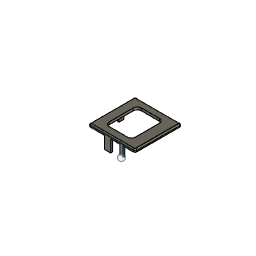
Lid (Autodesk Fusion 360 design; units mm, degrees)
Autodesk Fusion 360 part; units mm, degrees
ref_plane "WorkPlane1" through (0.6, 51.82, 34) normal (0, 0, 1) x (1, 0, 0)
sketch "Sketch1" plane through (0, 0, 34) normal (0, 0, 1) x (1, 0, 0)
  line L0 (53, -2) -> (1, -2)
  line L1 (-1, 0) -> (-1, 52)
  line L2 (1, 54) -> (53, 54)
  line L3 (55, 52) -> (55, 0)
  arc A0 (53, -2) -> (55, 0) centre (53, 0) ccw
  arc A1 (-1, 0) -> (1, -2) centre (1, 0) ccw
  arc A2 (1, 54) -> (-1, 52) centre (1, 52) ccw
  arc A3 (55, 52) -> (53, 54) centre (53, 52) ccw
  dimension "d94" = 2
  dimension "d95" = 2
  dimension "d96" = 2
  dimension "d97" = 2
  constraint horizontal L0
  constraint vertical L1
  constraint horizontal L2
  constraint vertical L3
  constraint tangent L0 A0
  constraint tangent L3 A0
  constraint tangent L0 A1
  constraint tangent L1 A1
  constraint tangent L2 A2
  constraint tangent L1 A2
  constraint tangent L2 A3
  constraint tangent L3 A3
  measures "d94" radius of A0
  measures "d95" radius of A1
  measures "d96" radius of A2
  measures "d97" radius of A3
extrude "Extrude1" add sketch "Sketch1" along normal blind 3
fillet "Fillet1" radius 1.5 8 edges at (55, 26, 37) (54.4142, 53.4142, 37) (27, 54, 37) (-0.4142, 53.4142, 37) (-1, 26, 37) (-0.4142, -1.4142, 37) (27, -2, 37) (54.4142, -1.4142, 37)
sketch "Sketch10" plane through (0, 0, 37) normal (0, 0, 1) x (-1, 0, 0)
  line L0 (-53.5, 0) -> (-53.5, -52)
  arc A0 (-53.5, -52) -> (-53, -52.5) centre (-53, -52) ccw
  line L1 (-53, -52.5) -> (-1, -52.5)
  arc A1 (-1, -52.5) -> (-0.5, -52) centre (-1, -52) ccw
  line L2 (-0.5, -52) -> (-0.5, 0)
  arc A2 (-0.5, 0) -> (-1, 0.5) centre (-1, 0) ccw
  line L3 (-1, 0.5) -> (-53, 0.5)
  arc A3 (-53, 0.5) -> (-53.5, 0) centre (-53, 0) ccw
  line L4 (-41.7153, -40.7644) -> (-41.7153, -11.7844) construction
  line L5 (-36.9153, -6.9844) -> (-14.9183, -6.9844) construction
  line L6 (-10, 0) -> (-10, -52.5) construction
  line L7 (-53.5, -45.7644) -> (-0.5, -45.7644) construction
  line L8 (-33.1772, -45.7644) -> (-36.8653, -45.7644) construction
  line L9 (-36.7153, -6.9844) -> (-15, -6.9844)
  line L10 (-10, -11.9844) -> (-10, -40.7644)
  line L11 (-15, -45.7644) -> (-36.7153, -45.7644)
  line L12 (-41.7153, -40.7644) -> (-41.7153, -11.9844)
  arc A4 (-15, -45.7644) -> (-10, -40.7644) centre (-15, -40.7644) ccw
  arc A5 (-41.7153, -40.7644) -> (-36.7153, -45.7644) centre (-36.7153, -40.7644) ccw
  arc A6 (-36.7153, -6.9844) -> (-41.7153, -11.9844) centre (-36.7153, -11.9844) ccw
  arc A7 (-10, -11.9844) -> (-15, -6.9844) centre (-15, -11.9844) ccw
  dimension "d123" = 5
  dimension "d124" = 5
  dimension "d125" = 5
  dimension "d126" = 5
  constraint coincident L1 L6.end
  constraint perpendicular L1 L6
  constraint coincident L0 L7.start
  constraint coincident L2 L7.end
  constraint perpendicular L2 L7
  constraint collinear L7 L8
  constraint horizontal L9
  constraint vertical L10
  constraint horizontal L11
  constraint vertical L12
  constraint tangent L10 A4
  constraint tangent L11 A4
  constraint tangent L11 A5
  constraint tangent L12 A5
  constraint tangent L9 A6
  constraint tangent L12 A6
  constraint tangent L9 A7
  constraint tangent L10 A7
  measures "d123" radius of A4
  measures "d124" radius of A5
  measures "d125" radius of A6
  measures "d126" radius of A7
extrude "Extrude2" cut sketch "Sketch10" against normal blind 3.25 contours L9 L10 L11 L12 A4 A5 A6 A7
sketch "Sketch11" plane through (0, 0, 34) normal (0, 0, -1) x (1, 0, 0)
  line L0 (10, -40.7644) -> (10, -11.9844)
  arc A0 (15, -6.9844) -> (10, -11.9844) centre (15, -11.9844) ccw
  line L1 (15, -6.9844) -> (36.7153, -6.9844)
  arc A1 (41.7153, -11.9844) -> (36.7153, -6.9844) centre (36.7153, -11.9844) ccw
  line L2 (41.7153, -11.9844) -> (41.7153, -40.7644)
  arc A2 (36.7153, -45.7644) -> (41.7153, -40.7644) centre (36.7153, -40.7644) ccw
  line L3 (36.7153, -45.7644) -> (15, -45.7644)
  arc A3 (10, -40.7644) -> (15, -45.7644) centre (15, -40.7644) ccw
  arc A4 (55, 0) -> (53, 2) centre (53, 0) ccw
  line L4 (53, 2) -> (1, 2)
  arc A5 (1, 2) -> (-1, 0) centre (1, 0) ccw
  line L5 (-1, 0) -> (-1, -52)
  arc A6 (-1, -52) -> (1, -54) centre (1, -52) ccw
  line L6 (1, -54) -> (53, -54)
  arc A7 (53, -54) -> (55, -52) centre (53, -52) ccw
  line L7 (55, -52) -> (55, 0)
  line L8 (53, -0.18) -> (26.8, -0.18) construction
  line L9 (0.6, -0.18) -> (0.6, -52) construction
  line L10 (0.6, -52) -> (53, -52) construction
  line L11 (53, -52) -> (53, -0.18) construction
  line L12 (26.8, -0.18) -> (0.6, -0.18) construction
  line L13 (18.2, 2) -> (18.2, -0.18)
  line L14 (25.8, 2) -> (25.8, -0.18)
  line L15 (36.7378, 2) -> (36.7378, -0.18)
  line L16 (40.4878, 2) -> (40.4878, -0.18)
  line L17 (-1, -39.0226) -> (0.6, -39.0226)
  line L18 (0.6, -39.0226) -> (0.6, -32.9226)
  line L19 (0.6, -32.9226) -> (-1, -32.9226)
  line L20 (-1, -32.9226) -> (-1, -39.0226)
  line L21 (-1.0059, -39.0226) -> (0.5941, -39.0226)
  line L22 (18.2, -0.18) -> (25.8, -0.18)
  line L23 (25.8, -0.18) -> (25.8, 2)
  line L24 (25.8, 2) -> (18.2, 2)
  line L25 (18.2, 2) -> (18.2, -0.18)
  line L26 (36.7378, -0.18) -> (40.4878, -0.18)
  line L27 (40.4878, -0.18) -> (40.4878, 2)
  line L28 (40.4878, 2) -> (36.7378, 2)
  line L29 (36.7378, 2) -> (36.7378, -0.18)
  point P0 (-1.0059, -32.9226)
  dimension "d129" = -2.18
  dimension "d131" = -2
  dimension "d136" = 3.75
  constraint perpendicular L9 L12
  constraint equal L8 L12
  constraint coincident L9.end L10.start
  constraint coincident L4 L13.start
  constraint coincident L12 L13.end
  constraint perpendicular L12 L13
  constraint coincident L4 L14.start
  constraint coincident L12 L14.end
  constraint perpendicular L12 L14
  constraint coincident L4 L15.start
  constraint coincident L8 L15.end
  constraint perpendicular L8 L15
  constraint coincident L4 L16.start
  constraint coincident L8 L16.end
  constraint perpendicular L8 L16
  constraint horizontal L17
  constraint vertical L18
  constraint horizontal L19
  constraint vertical L20
  constraint coincident L9 L18.end
  constraint coincident L5 L17.start
  constraint coincident L19 P0
  constraint coincident L17.start L21
  constraint horizontal L22
  constraint vertical L23
  constraint horizontal L24
  constraint vertical L25
  constraint horizontal L26
  constraint vertical L27
  constraint horizontal L28
  constraint vertical L29
  measures "d136" distance of L15.end L16.end
extrude "Extrude3" add sketch "Sketch11" along normal blind 12.6 contours L5 L17 L18 L19 L20 L21
extrude "Extrude4" add sketch "Sketch11" along normal blind 12.5 contours L4 L15 L16 L26 L27 L28 L29
sketch "Sketch2" plane through (0, -2, 0) normal (0, -1, 0) x (1, 0, 0)
  line L0 (53, 35.5) -> (1, 35.5)
  line L1 (1, 35.5) -> (1, 34)
  line L2 (1, 34) -> (36.7378, 34)
  line L3 (36.7378, 34) -> (36.7378, 21.5)
  line L4 (36.7378, 21.5) -> (40.4878, 21.5)
  line L5 (40.4878, 21.5) -> (40.4878, 34)
  line L6 (40.4878, 34) -> (53, 34)
  line L7 (53, 34) -> (53, 35.5)
  circle A0 centre (38.6128, 20.7133) radius 1.8901
extrude "Extrude6" add sketch "Sketch11" along normal blind 14.7 contours L4 L13 L14 L22 L23 L24 L25
extrude "Extrude7" cut sketch "Sketch2" against normal blind 2.5 contours L4 A0 picked at (38.4785, 21.9211)
extrude "Extrude5" [suppressed]
